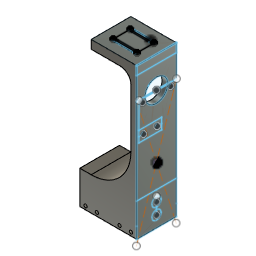
pendulum_shaft v2 (Autodesk Fusion 360 design; units mm, degrees)
Autodesk Fusion 360 part; units mm, degrees
sketch "Sketch1" plane through (0, 0, 0) normal (1, 0, 0) x (0, 1, 0)
  line L0 (-17.5916, -54.9708) -> (17.6035, 55.0079) construction
  line L1 (17.406, -55.0299) -> (-17.3965, 55) construction
  circle A0 centre (0, -30) radius 3.95
  line L2 (0, 55) -> (0.5, 55)
  line L3 (0, 55) -> (12.325, 55)
  line L4 (0, 55) -> (-12.325, 55)
  line L5 (-12.325, 55) -> (-12.325, 52)
  line L6 (12.325, 55) -> (12.325, 52)
  circle A1 centre (12.325, 52) radius 1.425
  circle A2 centre (-12.325, 52) radius 1.425
  circle A3 centre (0, -40) radius 3.95
  circle A4 centre (0, 55) radius 10
  line L7 (-15.3965, 54.9998) -> (-15.5, 32.25)
  circle A5 centre (-11.5, 27.45) radius 1.45
  line L8 (0, -30) -> (0, -40)
  line L9 (-17.3965, 55) -> (17.5, 55)
  line L10 (17.5, 55) -> (17.5, -40)
  line L11 (-17.3965, -40) -> (-17.3965, 55)
  line L12 (-17.3965, 55) -> (17.6035, 55)
  line L13 (17.6035, 55) -> (17.6035, 82.5)
  line L14 (17.6035, 82.5) -> (-17.3965, 82.5)
  line L15 (-17.3965, 82.5) -> (-17.3965, 55)
  line L16 (-17.3965, 82.5) -> (17.5, 82.5)
  line L17 (17.5, 82.5) -> (17.5, 75)
  line L18 (17.5, 75) -> (-17.3965, 75)
  line L19 (-17.3965, 75) -> (-17.3965, 82.5)
  line L20 (-15.5, 32.25) -> (4.5, 32.25)
  line L21 (4.5, 32.25) -> (4.5, 22.65)
  line L22 (4.5, 22.65) -> (-15.5, 22.65)
  line L23 (-15.5, 22.65) -> (-15.5, 32.25)
  circle A6 centre (0.5, 27.4838) radius 1.45
  line L24 (4.5, 27.45) -> (0.5, 27.45)
  line L25 (0.5, 27.45) -> (0.5, 27.4838)
  line L26 (-15.5, 27.45) -> (-11.5, 27.45)
  line L27 (0, -40) -> (0, -25.7392)
  line L28 (0, -20.7392) -> (-17.3965, -20.7392)
  line L29 (0, -20.7392) -> (17.5, -20.7392)
  line L30 (-17.3965, -40) -> (-17.3965, -50)
  line L31 (-17.3965, -50) -> (17.5, -50)
  line L32 (17.5, -50) -> (17.5, -40)
  dimension "d1" = 35
  dimension "d3" = 7.9
  dimension "d4" = 12.325
  dimension "d5" = 12.325
  dimension "d6" = 3
  dimension "d7" = 3
  dimension "d8" = 2.85
  dimension "d9" = 2.85
  dimension "d10" = 85
  dimension "d11" = 7.9
  dimension "d33" = 22.75
  dimension "d34" = 2
  dimension "d37" = 2.9
  dimension "d43" = 20
  dimension "d44" = 35
  dimension "d45" = 27.5
  dimension "d46" = 7.5
  dimension "d47" = 20
  dimension "d48" = 9.6
  dimension "d49" = 2.9
  dimension "d51" = 4
  dimension "d52" = 4
  dimension "d53" = 5
  dimension "d100" = 95
  constraint coincident L0 origin
  constraint coincident L1 origin
  constraint perpendicular L4 L5
  constraint perpendicular L3 L6
  constraint coincident L6.end A1.centre
  constraint coincident L5.end A2.centre
  constraint coincident L2.start L3.start
  constraint coincident A0.centre L8.start
  constraint horizontal L9
  constraint vertical L10
  constraint vertical L11
  constraint horizontal L12
  constraint vertical L13
  constraint horizontal L14
  constraint vertical L15
  constraint horizontal L16
  constraint vertical L17
  constraint horizontal L18
  constraint vertical L19
  constraint horizontal L20
  constraint vertical L21
  constraint horizontal L22
  constraint vertical L23
  constraint midpoint L21 L24.start
  constraint perpendicular L21 L24
  constraint coincident A6.centre L25.end
  constraint perpendicular L24 L25
  constraint midpoint L23 L26.start
  constraint perpendicular L23 L26
  constraint coincident A5.centre L26.end
  constraint coincident A3.centre L8.end
  constraint parallel L11 L27
  constraint coincident L11 L28.end
  constraint perpendicular L11 L28
  constraint coincident L10 L29.end
  constraint perpendicular L10 L29
  constraint parallel L11 L30
  constraint perpendicular L10 L31
  constraint perpendicular L31 L32
  measures "d1" distance of L0.end L1.end L2.end
  measures "d3" diameter of A0
  measures "d4" distance of L2.start L3.end
  measures "d5" distance of L2.start L4.end
  measures "d6" distance of L4.end L5.end
  measures "d7" distance of L3.end L6.end
  measures "d8" diameter of A1
  measures "d9" diameter of A2
  measures "d10" vertical distance of A0.centre L2.start
  measures "d11" diameter of A3
  measures "d33" distance of L7.start L7.end
  measures "d34" distance of L1.end L7.start
  measures "d37" diameter of A5
  measures "d43" diameter of A4
  measures "d44" distance of L1.end L12.end
  measures "d45" distance of L1.end L14.end
  measures "d46" distance of L14.end L18.end
  measures "d47" distance of L7.end L20.end
  measures "d48" distance of L7.end L22.end
  measures "d49" diameter of A6
  measures "d51" distance of L24.start L24.end
  measures "d52" distance of L26.start A5.centre
  measures "d53" distance of L27.end L28.start
  measures "d100" distance of A3.centre L9
extrude "Extrude8" add sketch "Sketch1" against normal blind 5 contours L2 L3 L4 A4 L9 L12 | L3 L4 A4 L9 L10 L11 L12 L28 L29 | A1 | A2 picked at (-6.6294, 55.4968) makes body 1
extrude "Extrude9" add sketch "Sketch1" against normal blind 40 contours L14 L15 L16 L17 L18 L19 bodies 1 makes body 2
extrude "Extrude10" add sketch "Sketch1" against normal blind 50 contours L10 L11 L28 L29 L30 L31 L32 bodies 1 2
extrude "Extrude11" add sketch "Sketch1" against normal blind 5 contours A0 L8 L27 | A0 L8 L27 | A3 bodies 2 1
extrude "Extrude12" add sketch "Sketch1" against normal blind 5 contours L20 L21 L22 L23 bodies 2 1
sketch "Sketch4" plane through (0, 0, 82.5) normal (0, 0, 1) x (-1, 0, 0)
  line L0 (0, 17.3965) -> (0, -17.5)
  line L1 (0, -17.5) -> (40, -17.5)
  line L2 (40, -17.5) -> (40, 17.3965)
  line L3 (40, 17.3965) -> (0, 17.3965)
  line L4 (30.5, -7.5) -> (9.5, -7.5)
  line L5 (9.5, -7.5) -> (9.5, 7.5)
  line L6 (9.5, 7.5) -> (30.5, 7.5)
  line L7 (30.5, 7.5) -> (30.5, -7.5)
  circle A0 centre (30.5, -7.5) radius 1.425
  circle A1 centre (9.5, -7.5) radius 1.425
  circle A2 centre (9.5, 7.5) radius 1.425
  circle A3 centre (30.5, 7.5) radius 1.425
  line L8 (30.5086, -8.925) -> (9.5, -8.925)
  line L9 (9.5, -8.925) -> (9.5, -6.075)
  line L10 (9.5, -6.075) -> (30.5086, -6.075)
  line L11 (30.5086, -6.075) -> (30.5086, -8.925)
  line L12 (30.5, 6.075) -> (9.5, 6.075)
  line L13 (9.5, 6.075) -> (9.5, 8.925)
  line L14 (9.5, 8.925) -> (30.5, 8.925)
  line L15 (30.5, 8.925) -> (30.5, 6.075)
  line L16 (29.075, 7.5) -> (27.575, 7.5)
  line L17 (10.925, 7.5) -> (12.425, 7.5)
  line L18 (29.075, -7.5) -> (27.575, -7.5)
  line L19 (10.925, -7.5) -> (12.425, -7.5)
  line L20 (27.575, -7.5) -> (27.575, -6.075)
  line L21 (27.575, -7.5) -> (27.575, -7.7664)
  line L22 (27.575, -7.7664) -> (27.575, -8.925)
  line L23 (12.425, -8.925) -> (12.425, -6.075)
  line L24 (10.9687, 6.075) -> (10.9687, 8.925)
  line L25 (12.425, 7.5) -> (12.425, 7.1994)
  line L26 (12.425, 7.1994) -> (12.425, 6.075)
  line L27 (12.425, 7.5) -> (12.425, 8.925)
  line L28 (27.575, 7.5) -> (27.575, 6.075)
  line L29 (27.575, 7.5) -> (27.575, 8.925)
  dimension "d68" = 21
  dimension "d69" = 15
  dimension "d70" = 10
  dimension "d71" = 9.5
  dimension "d72" = 2.85
  dimension "d73" = 2.85
  dimension "d74" = 2.85
  dimension "d75" = 2.85
  dimension "d76" = 1.5
  dimension "d77" = 1.5
  dimension "d78" = 1.5
  dimension "d79" = 1.5
  constraint horizontal L4
  constraint vertical L5
  constraint horizontal L6
  constraint vertical L7
  constraint coincident L4.start L7.end
  constraint coincident L4.end L5.start
  constraint coincident L5.end L6.start
  constraint coincident L6.end L7.start
  constraint horizontal L8
  constraint vertical L9
  constraint horizontal L10
  constraint vertical L11
  constraint coincident A1 L9.end
  constraint coincident L5 L9.end
  constraint coincident A0 L8.start
  constraint horizontal L12
  constraint vertical L13
  constraint horizontal L14
  constraint vertical L15
  constraint coincident A2 L13.end
  constraint coincident L7 L12.start
  constraint coincident A3 L12.start
  constraint coincident A3 L16.start
  constraint coincident L6 L16.start
  constraint coincident L6 L16.end
  constraint coincident A2 L17.start
  constraint coincident L6 L17.start
  constraint perpendicular L13 L17
  constraint coincident L4 L18.start
  constraint coincident A0 L18.start
  constraint perpendicular L7 L18
  constraint coincident A1 L19.start
  constraint coincident L4 L19.start
  constraint parallel L4 L19
  constraint coincident L10 L20.end
  constraint perpendicular L10 L20
  constraint perpendicular L4 L21
  constraint coincident L8 L22.end
  constraint perpendicular L8 L22
  constraint coincident L8 L23.start
  constraint coincident L10 L23.end
  constraint perpendicular L10 L23
  constraint coincident L12 L24.start
  constraint coincident L14 L24.end
  constraint perpendicular L14 L24
  constraint perpendicular L17 L25
  constraint coincident L12 L26.end
  constraint perpendicular L12 L26
  constraint coincident L14 L27.end
  constraint perpendicular L14 L27
  constraint coincident L12 L28.end
  constraint perpendicular L12 L28
  constraint coincident L14 L29.end
  constraint perpendicular L14 L29
  measures "d68" distance of L4.start L4.end
  measures "d69" distance of L4.start L6.end
  measures "d70" distance of L1 L4
  measures "d71" distance of L2 L7
  measures "d72" diameter of A0
  measures "d73" diameter of A1
  measures "d74" diameter of A2
  measures "d75" diameter of A3
  measures "d76" distance of L16.start L16.end
  measures "d77" distance of L17.start L17.end
  measures "d78" distance of L18.start L18.end
  measures "d79" distance of L19.start L19.end
extrude "Extrude13" add sketch "Sketch4" against normal blind 3 separate body contours L4 L8 L21 L22 L23 | L4 L10 L20 L23 | L6 L12 L25 L26 L28 | L6 L14 L27 L29 makes body 3 at (-17.475, 6.075, 80.5) makes body 4 at (-22.525, -6.075, 80.5)
extrude "Extrude14" cut sketch "Sketch4" against normal blind 5 contours L4 L7 A0 L10 L11 | L4 L7 A0 | A0 L11 | L6 L7 A3 L15 | L7 A3 L15 | L6 A3 L15 | L4 A1 L9 | L4 L5 A1 L9 | L5 A1 L9 | L5 A2 L13 | L5 L6 A2 L13 | L6 A2 L13 bodies 1 2
extrude "Extrude15" cut sketch "Sketch4" against normal blind 3 contours L4 L8 L21 L22 L23 | L4 L10 L20 L23 | L6 L12 L25 L26 L28 | L6 L14 L27 L29 bodies 2 1
extrude "Extrude16" cut 1 faces at (-22.525, -7.025, 82.5) along direction (0, 0, -1) blind 3 on bodies 4 bodies 4
extrude "Extrude17" cut 1 faces at (-17.475, 7.025, 82.5) along direction (0, 0, -1) blind 3 on bodies 3 bodies 3
extrude "Extrude18" add sketch "Sketch1" against normal blind 10 contours A0 L8 L27 | A0 L8 L27 | L2 L3 L4 A4 L9 L12 | L3 L4 A4 L9 L10 L11 L12 L28 L29 | L10 L11 L28 L29 L30 L31 L32 | A1 | A2 | A3 | A5 | L20 L21 L22 L23 | A6 picked at (-3.745, 49.5071) bodies 1 2 3 4
extrude "Extrude19" cut sketch "Sketch1" against normal blind 10 contours L2 L3 L4 A4 L9 L12 picked at (-3.745, 49.5071) bodies 2 1
extrude "Extrude20" cut 1 faces at (-10, 0.2836, 1.1832) along direction (1, 0, 0) blind 5 on bodies 1 bodies 1 2
extrude "Extrude21" add sketch "Sketch1" against normal blind 5 contours L3 L4 A4 L9 L12 L13 L14 L15 L17 L18 bodies 1 2
extrude "Extrude22" cut sketch "Sketch1" against normal blind 5 contours L2 L3 L4 A4 L9 L12 picked at (-6.6294, 55.4968) bodies 1
extrude "Extrude23" cut sketch "Sketch1" against normal blind 5 contours A1 | A2 bodies 1
sketch "Sketch5" plane through (0, 17.5, 0) normal (0, 1, 0) x (-1, 0, 0)
  line L0 (50, -20.7392) -> (5, -20.7392)
  line L1 (5, -20.7392) -> (5, 55)
  line L2 (5, 55) -> (0, 55)
  line L3 (0, 55) -> (0, -50)
  line L4 (0, -50) -> (50, -50)
  line L5 (50, -50) -> (50, -20.7392)
  circle A0 centre (5, -47) radius 1.425
  line L6 (0, -50) -> (0, -40)
  circle A1 centre (15, -47) radius 1.425
  circle A2 centre (35, -47) radius 1.425
  circle A3 centre (45, -47) radius 1.425
  dimension "d111" = 2.85
  dimension "d112" = 5
  dimension "d113" = 2.85
  dimension "d114" = 2.85
  dimension "d115" = 2.85
  dimension "d116" = 5
  dimension "d117" = 10
  dimension "d118" = 20
  dimension "d119" = 10
  dimension "d120" = 3
  dimension "d121" = 3
  dimension "d122" = 3
  dimension "d123" = 3
  measures "d111" diameter of A0
  measures "d112" distance of A0.centre L6
  measures "d113" diameter of A1
  measures "d114" diameter of A2
  measures "d115" diameter of A3
  measures "d116" distance of L5 A3.centre
  measures "d117" distance of A2.centre A3.centre
  measures "d118" distance of A1.centre A2.centre
  measures "d119" distance of A0.centre A1.centre
  measures "d120" distance of L4 A0.centre
  measures "d121" distance of L4 A1.centre
  measures "d122" distance of L4 A2.centre
  measures "d123" distance of L4 A3.centre
extrude "Extrude24" cut sketch "Sketch5" against normal blind 35 contours A0 | A1 | A2 | A3 bodies 1
fillet "Fillet6" radius 9.5 1 edges at (-5, 0.0518, 75) on bodies 1
fillet "Fillet7" radius 35 1 edges at (-5, 0.0518, -20.7392) on bodies 1
equation "d4 = ( 24.65 / 2 ) * 1 mm"
equation "d5 = ( 24.65 / 2 ) * 1 mm"
